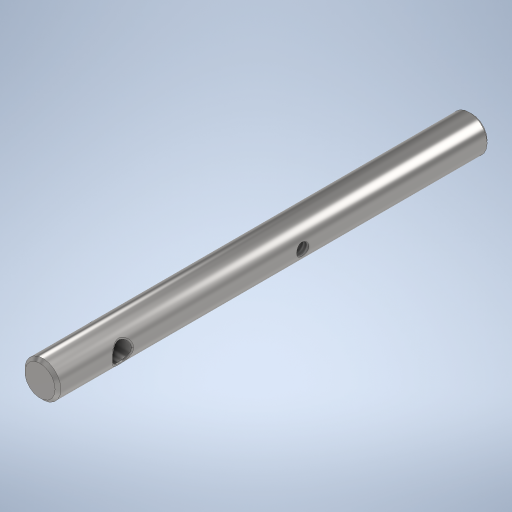
# Autodesk Inventor part: Carriage Axle V1
Saved by Autodesk Inventor 2023 (Build 270158000, 158)
## iProperties
Created: 2023-02-13
Part Number: Carriage Axle V1
Material: Stainless Steel
Document SubType Name: Modeling
Designer: mbear
Density: 8 g/cm^3
Appearance: Semi-Polished
Author: mbear
Autodesk Inventor part; units mm, degrees
ref_plane "XZ Plane" through (0, 0, 0) normal (0, 1, 0) x (-1, 0, 0)
ref_plane "XY Plane" through (0, 0, 0) normal (0, 0, 1) x (1, 0, 0)
sketch "Sketch1" plane through (0, 0, 0) normal (0, 0, 1) x (1, 0, 0)
  circle A0 centre (0, 0) radius 3.175
  dimension "d0" = 6.35
  constraints: 1 centre point, 1 coincident
  measures "d0" diameter of A0
extrude "Extrusion1" add sketch "Sketch1" against normal blind 76.2
chamfer "Chamfer1" distance 0.508 angle 45 2 edges at (-3.175, 0, 0) (-3.175, 0, -76.2)
ref_plane "Work Plane1" through (3.175, 0, 0) normal (1, 0, 0) x (0, 1, 0)
sketch "Sketch2" plane through (3.175, 0, 0) normal (1, 0, 0) x (0, 1, 0)
  circle A0 centre (0, -11.43) radius 2.5906
  point P0 (0, 0)
  dimension "d7" = 11.43
  dimension "d8" = 5.1811
  constraints: 1 centre point, 1 vertical alignment
  measures "d7" distance of A0.centre point (0, 0)
  measures "d8" diameter of A0
hole "Hole1" at (3.175, 0, -11.43) direction (-1, 0, 0) diameter 3.4 depth 25.4 tip angle 118 clearance for "Socket Head Cap Screw" size "M3" standard "Ansi Metric M Profile"
fillet "Fillet1" radius 0.2 3 edges at (2.6815, 1.7, -11.4301) (2.6815, -1.7, -11.4299) (-3.175, 0.0097, -9.73)
sketch "Sketch3" plane through (3.175, 0, 0) normal (1, 0, 0) x (0, 1, 0)
  circle A0 centre (0, -43.18) radius 1.738
  point P0 (0, 0)
  dimension "d17" = 43.18
  constraints: 1 centre point
  measures "d17" distance of point (0, 0) A0.centre
hole "Hole2" at (3.175, 0, -43.18) direction (-1, 0, 0) diameter 2.1565 depth 3.175 tip angle 118 thread size "4-40 UNC" class "2B" standard "ANSI Unified Screw Threads"
body "Solid1"
